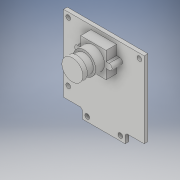
# Autodesk Inventor part: pixy-cam
Saved by Autodesk Inventor 2018 (Build 220112000, 112)
## iProperties
Created: 2017-10-10
Part Number: pixy-cam
Material: Generic
Document SubType Name: Modeling
Designer: leo2a
Density: 1 g/cm^3
Appearance: Default
Author: leo2a
Autodesk Inventor part; units mm, degrees
ref_plane "YZ Plane" through (0, 0, 0) normal (1, 0, 0) x (0, 1, 0)
ref_plane "XZ Plane" through (0, 0, 0) normal (0, 1, 0) x (-1, 0, 0)
ref_plane "XY Plane" through (0, 0, 0) normal (0, 0, 1) x (1, 0, 0)
sketch "Sketch1" plane through (0, 0, 0) normal (0, 0, 1) x (1, 0, 0)
  line L0 (26.924, 25.4) -> (26.924, -25.4)
  line L1 (26.924, -25.4) -> (15.494, -25.4)
  line L2 (14.224, -26.67) -> (14.224, -31.75)
  line L3 (14.224, -31.75) -> (0, -31.75)
  line L4 (26.924, 25.4) -> (0, 25.4)
  line L5 (-26.924, 25.4) -> (-26.924, -25.4)
  line L6 (-26.924, -25.4) -> (-15.494, -25.4)
  line L7 (-14.224, -26.67) -> (-14.224, -31.75)
  line L8 (-14.224, -31.75) -> (0, -31.75)
  line L9 (-26.924, 25.4) -> (0, 25.4)
  line L10 (-15.494, -25.4) -> (-14.224, -26.67)
  line L11 (14.224, -26.67) -> (15.494, -25.4)
  point P0 (0, 0)
  point P1 (14.224, -25.4)
  point P2 (-14.224, -25.4)
  constraints: 24 end point, 4 point on line, 3 perpendicular, 1 horizontal
extrude "Extrusion1" add sketch "Sketch1" along normal blind 2.54
sketch "Sketch2" plane through (0, 0, 2.54) normal (0, 0, 1) x (1, 0, 0)
  point P0 (0, 0)
  point P1 (26.924, 25.4)
  point P2 (-23.749, 22.225)
  point P3 (23.749, 22.225)
  point P4 (-23.749, -17.272)
  point P5 (-11.049, -28.575)
  point P6 (11.049, -28.575)
hole "Hole1" at (-23.749, 22.225, 2.54) at (23.749, 22.225, 2.54) at (-23.749, -17.272, 2.54) at (-11.049, -28.575, 2.54) at (11.049, -28.575, 2.54) direction (0, 0, -1) diameter 3.175 end through all
sketch "Sketch3" plane through (0, 0, 2.54) normal (0, 0, 1) x (1, 0, 0)
  line L0 (26.924, 25.4) -> (-26.924, 25.4) projected
  line L1 (0, 25.4) -> (0, 22.86)
  line L2 (0, 22.86) -> (0, 14.36)
  line L3 (-8.5, 5.86) -> (8.5, 5.86)
  line L4 (8.5, 5.86) -> (8.5, 22.86)
  line L5 (8.5, 22.86) -> (-8.5, 22.86)
  line L6 (-8.5, 22.86) -> (-8.5, 5.86)
  line L7 (-8.5, 5.86) -> (8.5, 22.86) construction
  line L8 (8.5, 5.86) -> (-8.5, 22.86) construction
  point P0 (0, 0)
  dimension "d27" = 2.54
  dimension "d28" = 8.5
  dimension "d29" = 17
  constraints: 16 end point, 3 midpoint, 2 parallel, 2 vertical, 1 horizontal, 1 perpendicular
  measures "d27" distance of L1.start L1.end
  measures "d28" distance of L1.end L2.end
  measures "d29" distance of L3.start L3.end
extrude "Extrusion2" add sketch "Sketch3" along normal blind 7
sketch "Sketch4" plane through (0, 0, 9.54) normal (0, 0, 1) x (1, 0, 0)
  circle A0 centre (0, 14.36) radius 7.5
  circle A1 centre (0, 14.36) radius 6
  point P0 (0, 0)
  dimension "d32" = 15
  dimension "d33" = 12
  constraints: 2 centre point, 1 coincident
  measures "d32" diameter of A0
  measures "d33" diameter of A1
extrude "Extrusion3" add sketch "Sketch4" along normal blind 6
sketch "Sketch5" plane through (0, 14.36, 15.54) normal (0, 0, 1) x (1, 0, 0)
  circle A0 centre (0, 0) radius 6
  point P0 (0, -14.36)
  constraints: 1 centre point
extrude "Extrusion4" add sketch "Sketch5" along normal blind 5
sketch "Sketch6" plane through (0, 14.36, 20.54) normal (0, 0, 1) x (1, 0, 0)
  circle A0 centre (0, 0) radius 7
  point P0 (0, -14.36)
  dimension "d38" = 14
  constraints: 1 centre point
  measures "d38" diameter of A0
extrude "Extrusion5" add sketch "Sketch6" along normal blind 3
sketch "Sketch7" plane through (0, 0, 2.54) normal (0, 0, 1) x (1, 0, 0)
  line L0 (-8.5, 22.86) -> (-8.5, 5.86) projected
  line L1 (-8.5, 14.36) -> (-10.5, 14.36)
  circle A0 centre (-10.5, 14.36) radius 2
  line L2 (-10.5, 16.36) -> (-8.5, 16.36)
  line L3 (-10.5, 12.36) -> (-8.5, 12.36)
  point P0 (0, 0)
  dimension "d41" = 2
  constraints: 6 end point, 3 point on circle, 2 perpendicular, 2 point on line, 1 centre point, 1 coincident, 1 horizontal, 1 midpoint
  measures "d41" distance of L1.start L1.end
extrude "Extrusion6" add sketch "Sketch7" along normal up to surface (7 mm away)
mirror "Mirror1" about plane through (0, 0, 0) normal (1, 0, 0) of "Extrusion6"
body "Solid1"
